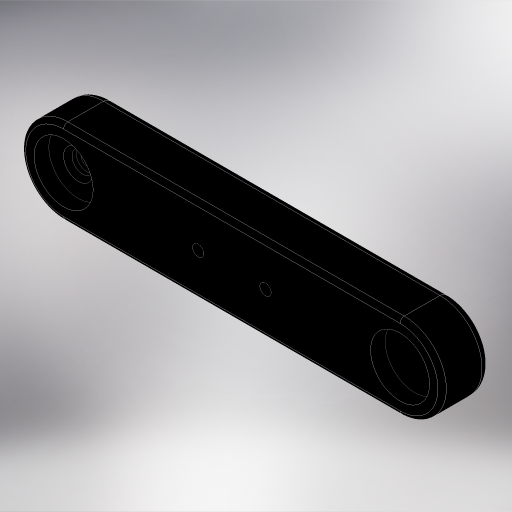
# Autodesk Inventor part: Plate E
Saved by Autodesk Inventor 2024 (Build 280153000, 153)
## iProperties
Created: 2023-12-17
Part Number: Plate E
Material: Generic
Document SubType Name: Modeling
Designer: aaron
Density: 1 g/cm^3
Appearance: Default
Author: aaron
Autodesk Inventor part; units mm, degrees
ref_plane "YZ Plane" through (0, 0, 0) normal (1, 0, 0) x (0, 1, 0)
ref_plane "XZ Plane" through (0, 0, 0) normal (0, 1, 0) x (-1, 0, 0)
ref_plane "XY Plane" through (0, 0, 0) normal (0, 0, 1) x (1, 0, 0)
sketch "Sketch1" plane through (0, 0, 0) normal (0, 0, 1) x (1, 0, 0)
  circle A0 centre (0, 0) radius 15.875
  line L0 (0, 0) -> (-127, 0)
  circle A1 centre (-127, 0) radius 15.875
  line L1 (-127, 15.875) -> (0, 15.875)
  line L2 (0, -15.875) -> (-127, -15.875)
  circle A2 centre (-127, 0) radius 2.1082
  dimension "d0" = 31.75
  dimension "d1" = 127
  dimension "d2" = 31.75
  dimension "d3" = 4.2164
  constraints: 6 end point, 4 point on circle, 3 centre point, 3 coincident, 2 horizontal, 1 tangent
  measures "d0" diameter of A0
  measures "d1" distance of L0.start L0.end
  measures "d2" diameter of A1
  measures "d3" diameter of A2
extrude "Extrusion1" add sketch "Sketch1" along normal blind 3.175
sketch "Sketch2" plane through (0, 0, 0) normal (0, 0, -1) x (-1, 0, 0)
  arc A0 (127, -15.875) -> (127, 15.875) centre (127, 0) ccw projected
  line L0 (0, 15.875) -> (127, 15.875) projected
  arc A1 (0, 15.875) -> (0, -15.875) centre (0, 0) ccw projected
  line L1 (127, -15.875) -> (0, -15.875) projected
  circle A2 centre (127, 0) radius 2.1082 projected
  line L2 (130.175, -3.175) -> (123.825, -3.175)
  line L3 (123.825, -3.175) -> (123.825, 3.175)
  line L4 (123.825, 3.175) -> (130.175, 3.175)
  line L5 (130.175, 3.175) -> (130.175, -3.175)
  line L6 (130.175, -3.175) -> (123.825, 3.175) construction
  line L7 (123.825, -3.175) -> (130.175, 3.175) construction
  dimension "d25" = 6.35
  dimension "d26" = 6.35
  constraints: 12 end point, 2 midpoint, 2 parallel, 1 horizontal, 1 perpendicular
  measures "d25" distance of L3.end L4.end
  measures "d26" distance of L2.end L3.end
extrude "Extrusion2" add sketch "Sketch2" along normal blind 6.35 contours L1 A1 L0 A0
fillet "Fillet1" radius 3.175 4 edges at (15.875, 0, -6.35) (-63.5, -15.875, -6.35) (-142.875, 0, -6.35) (-63.5, 15.875, -6.35)
sketch "Sketch3" plane through (0, 0, 3.175) normal (0, 0, 1) x (1, 0, 0)
  arc A0 (-127, 15.875) -> (-127, -15.875) centre (-127, 0) ccw projected
  line L0 (-127, -15.875) -> (0, -15.875) projected
  arc A1 (0, -15.875) -> (0, 15.875) centre (0, 0) ccw projected
  line L1 (0, 15.875) -> (-127, 15.875) projected
  circle A2 centre (-127, 0) radius 2.1082 projected
  circle A3 centre (-127, 0) radius 3.9688
  dimension "d10" = 7.9375
  constraints: 1 centre point, 1 coincident
  measures "d10" diameter of A3
extrude "Extrusion3" add sketch "Sketch3" along normal blind 3.175 contours L1 A1 L0 A0
sketch "Sketch4" plane through (0, 0, 6.35) normal (0, 0, 1) x (1, 0, 0)
  line L0 (-127, -15.875) -> (0, -15.875) projected
  arc A0 (0, -15.875) -> (0, 15.875) centre (0, 0) ccw projected
  line L1 (0, 15.875) -> (-127, 15.875) projected
  arc A1 (-127, 15.875) -> (-127, -15.875) centre (-127, 0) ccw projected
  circle A2 centre (-127, 0) radius 3.9688 projected
  circle A3 centre (-127, 0) radius 2.1082 projected
  circle A4 centre (-127, 0) radius 11.1125
  circle A5 centre (0, 0) radius 11.1125
  dimension "d13" = 22.225
  dimension "d14" = 22.225
  constraints: 2 centre point, 2 coincident
  measures "d13" diameter of A4
  measures "d14" diameter of A5
extrude "Extrusion4" add sketch "Sketch4" along normal blind 5.5372 contours A1 L1 A0 L0
sketch "Sketch5" plane through (0, 0, 11.8872) normal (0, 0, 1) x (1, 0, 0)
  circle A0 centre (-76.2, 0) radius 2.1082
  circle A1 centre (-50.8, 0) radius 2.1082
  circle A2 centre (-127, 0) radius 2.1082 projected
  point P0 (0, 0)
  dimension "d17" = 4.2164
  dimension "d18" = 4.2164
  dimension "d19" = 50.8
  dimension "d20" = 50.8
  constraints: 2 centre point
  measures "d17" diameter of A0
  measures "d18" diameter of A1
  measures "d19" distance of point (0, 0) A1.centre
  measures "d20" distance of A2.centre A0.centre
extrude "Extrusion5" cut sketch "Sketch5" against normal blind 25.4 contours A0 | A1
fillet "Fillet2" radius 1.5875 4 edges at (-142.875, 0, 11.8872) (-63.5, -15.875, 11.8872) (15.875, 0, 11.8872) (-63.5, 15.875, 11.8872)
fillet "Fillet3" radius 1.5875 1 edges at (-130.9688, 0, 6.35)
body "Solid1"
